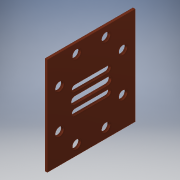
# Autodesk Inventor part: Valve Plate
Saved by Autodesk Inventor 2017 (Build 210142000, 142)
## iProperties
Created: 2018-11-01
Part Number: Valve Plate
Material: Copper, Alloy
Document SubType Name: Modeling
Designer: 623516
Density: 8.92 g/cm^3
Appearance: Copper - Satin
Author: 623516
Autodesk Inventor part; units mm, degrees
ref_plane "YZ Plane" through (0, 0, 0) normal (1, 0, 0) x (0, 1, 0)
ref_plane "XZ Plane" through (0, 0, 0) normal (0, 1, 0) x (-1, 0, 0)
ref_plane "XY Plane" through (0, 0, 0) normal (0, 0, 1) x (1, 0, 0)
sketch "Sketch1" plane through (0, 0, 0) normal (1, 0, 0) x (0, 1, 0)
  line L0 (0, 0) -> (40, 0)
  line L1 (40, 0) -> (40, -36)
  line L2 (40, -36) -> (0, -36)
  line L3 (0, -36) -> (0, 0)
  line L4 (20, -7.186) -> (4, -7.186) construction
  line L5 (4, -18) -> (4, -12) construction
  line L6 (4, -12) -> (8.3258, -12) construction
  line L7 (4, -18) -> (4, -24) construction
  circle A0 centre (4, -12) radius 1.75
  circle A1 centre (4, -24) radius 1.75
  line L8 (20, -7.186) -> (36, -7.186) construction
  line L9 (36, -18) -> (36, -12) construction
  line L10 (36, -18) -> (36, -24) construction
  circle A2 centre (36, -12) radius 1.75 construction
  circle A3 centre (36, -12) radius 1.75
  circle A4 centre (36, -24) radius 1.75
  line L11 (20, -4.4458) -> (12, -4.4458) construction
  line L12 (12, -18) -> (12, -5) construction
  line L13 (12, -18) -> (12, -31) construction
  circle A5 centre (12, -5) radius 1.75 construction
  circle A6 centre (12, -5) radius 1.75
  circle A7 centre (12, -31) radius 1.75
  line L14 (20, -5) -> (28, -5) construction
  circle A8 centre (28, -5) radius 1.75 construction
  circle A9 centre (28, -5) radius 1.75
  line L15 (28, -5) -> (28, -18) construction
  line L16 (28, -18) -> (28, -31) construction
  circle A10 centre (28, -31) radius 1.75 construction
  circle A11 centre (28, -31) radius 1.75
  line L17 (20, 0) -> (20, -36) construction
  line L18 (21.5, -18) -> (21.5, -11.25) construction
  line L19 (21.5, -11.25) -> (20, -11.25) construction
  line L20 (18.5, -11.25) -> (20, -11.25) construction
  line L21 (21.5, -11.25) -> (18.5, -11.25)
  line L22 (18.5, -24.75) -> (21.5, -24.75)
  line L23 (21.5, -11.25) -> (21.5, 28.048) construction
  line L24 (18.5, -11.25) -> (18.5, 31.5253) construction
  arc A12 (21.5, -11.25) -> (18.5, -11.25) centre (20, -11.25) ccw construction
  arc A13 (18.5, -24.75) -> (21.5, -24.75) centre (20, -24.75) ccw construction
  arc A14 (21.5, -11.25) -> (18.5, -11.25) centre (20, -11.25) ccw
  arc A15 (18.5, -24.75) -> (21.5, -24.75) centre (20, -24.75) ccw
  line L25 (21.5, -11.25) -> (21.5, -24.75)
  line L26 (18.5, -24.75) -> (18.5, -11.25)
  line L27 (21.5, -15) -> (23, -15) construction
  line L28 (23, -11.25) -> (23, -24.75) construction
  line L29 (23, -24.75) -> (25.5, -24.75) construction
  line L30 (25.5, -24.75) -> (25.5, -11.25) construction
  line L31 (25.5, -11.25) -> (23, -11.25) construction
  line L32 (25.5, -11.25) -> (25.5, -24.75)
  line L33 (23, -11.25) -> (23, -24.75)
  arc A16 (25.5, -11.25) -> (23, -11.25) centre (24.25, -11.25) ccw
  arc A17 (23, -24.75) -> (25.5, -24.75) centre (24.25, -24.75) ccw
  line L34 (18.5, -11.25) -> (17, -11.25) construction
  line L35 (17, -11.25) -> (17, -92.3561) construction
  line L36 (14.5, -11.25) -> (14.5, -24.75) construction
  line L37 (17, -11.25) -> (17, -24.75)
  line L38 (14.5, -24.75) -> (14.5, -11.25)
  arc A18 (17, -11.25) -> (14.5, -11.25) centre (15.75, -11.25) ccw
  arc A19 (14.5, -24.75) -> (17, -24.75) centre (15.75, -24.75) ccw
  line L39 (40, -18) -> (-21.6242, -18) construction
  dimension "d0" = 40
  dimension "d1" = 36
  dimension "d5" = 16
  dimension "d6" = 6
  dimension "d7" = 6
  dimension "d8" = 3.5
  dimension "d9" = 3.5
  dimension "d13" = 16
  dimension "d14" = 6
  dimension "d15" = 6
  dimension "d16" = 3.5
  dimension "d17" = 3.5
  dimension "d19" = 8
  dimension "d20" = 13
  dimension "d21" = 13
  dimension "d22" = 3.5
  dimension "d23" = 3.5
  dimension "d25" = 8
  dimension "d26" = 3.5
  dimension "d27" = 13
  dimension "d28" = 3.5
  dimension "d48" = 6.75
  dimension "d73" = 11.25
  dimension "d74" = 13.5
  dimension "d75" = 18.5
  dimension "d77" = 1.5
  dimension "d78" = 2.5
  dimension "d84" = 1.5
  dimension "d85" = 2.5
  dimension "d86" = 2.5
  dimension "d92" = 8
  dimension "d93" = 8
  dimension "d94" = 13
  constraints: 80 end point, 20 centre point, 17 tangent, 16 point on circle, 12 coincident, 10 parallel, 9 perpendicular, 5 horizontal, 5 point on line, 4 equal radius, 4 vertical, 3 collinear, 3 midpoint
  measures "d0" distance of L1.end L2.end
  measures "d1" distance of L0.end L1.end
  measures "d5" distance of L4.start L4.end
  measures "d6" distance of L5.start L5.end
  measures "d7" distance of L5.start L7.end
  measures "d8" diameter of A0
  measures "d9" diameter of A1
  measures "d13" distance of L4.start L8.end
  measures "d14" distance of L9.start L9.end
  measures "d15" distance of L9.start L10.end
  measures "d16" diameter of A2
  measures "d17" diameter of A4
  measures "d19" distance of L11.start L11.end
  measures "d20" distance of L12.start L12.end
  measures "d21" distance of L12.start L13.end
  measures "d22" diameter of A5
  measures "d23" diameter of A7
  measures "d25" distance of L14.start L14.end
  measures "d26" diameter of A8
  measures "d27" distance of L15.end L16.end
  measures "d28" diameter of A10
  measures "d48" distance of L18.start L18.end
  measures "d73" distance from line of L2 A13.centre
  measures "d74" distance of L18.end L22.end
  measures "d75" distance between parallel lines of L1 L25
  measures "d77" distance of L27.start L27.end
  measures "d78" distance of L28.end L29.end
  measures "d84" distance of L21.end L34.end
  measures "d85" distance of L34.end L36.start
  measures "d86" distance of L36.end L37.end
  measures "d92" distance from line of L16.end L17
  measures "d93" distance from line of L13.end L17
  measures "d94" distance from line of L39 L16.end
extrude "Extrusion3" add sketch "Sketch1" along normal blind 1
fillet "Fillet1" radius 0.1 4 edges at (0, 20, -36) (0, 40, -18) (0, 20, 0) (0, 0, -18)
body "Solid3"
